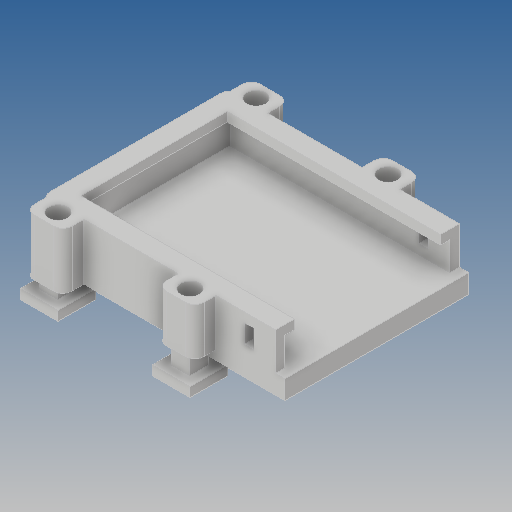
# Autodesk Inventor part: DC-DC корпус
Saved by Autodesk Inventor 2020 (Build 240168000, 168)
## iProperties
Created: 2020-03-21
Part Number: DC-DC корпус
Material: Типовые
Document SubType Name: Modeling
Designer: Iliga
Density: 1 g/cm^3
Appearance: По умолчанию
Author: Iliga
Autodesk Inventor part; units mm, degrees
ref_plane "YZ Plane" through (0, 0, 0) normal (1, 0, 0) x (0, 1, 0)
ref_plane "XZ Plane" through (0, 0, 0) normal (0, 1, 0) x (-1, 0, 0)
ref_plane "XY Plane" through (0, 0, 0) normal (0, 0, 1) x (1, 0, 0)
sketch "Эскиз1" plane through (0, 0, 0) normal (0, 1, 0) x (-1, 0, 0)
  line L0 (-11.5, 8.75) -> (11.5, 8.75)
  line L1 (11.5, 8.75) -> (11.5, -8.75)
  line L2 (11.5, -8.75) -> (-11.5, -8.75)
  line L3 (-11.5, -8.75) -> (-11.5, 8.75)
  line L4 (-11.5, 8.75) -> (11.5, -8.75) construction
  line L5 (11.5, 8.75) -> (-11.5, -8.75) construction
  line L6 (-12.8143, 9.75) -> (12.8143, 9.75)
  line L7 (12.8143, 9.75) -> (12.8143, -9.75)
  line L8 (12.8143, -9.75) -> (-12.8143, -9.75)
  line L9 (-12.8143, -9.75) -> (-12.8143, 9.75)
  line L10 (-12.8143, 9.75) -> (12.8143, -9.75) construction
  line L11 (12.8143, 9.75) -> (-12.8143, -9.75) construction
  point P0 (0, 0)
  dimension "d0" = 23
  dimension "d1" = 17.5
  dimension "d2" = 1
  constraints: 24 end point, 4 midpoint, 4 parallel, 2 horizontal, 2 perpendicular, 1 point on line
  measures "d0" distance of L1.end L2.end
  measures "d1" distance of L0.end L1.end
  measures "d2" distance between parallel lines of L8 L2
extrude "Выдавливание1" add sketch "Эскиз1" against normal blind 1 contours L0 L1 L2 L3 | L6 L7 L8 L9
extrude "Выдавливание2" add sketch "Эскиз1" along normal blind 3
sketch "Эскиз2" plane through (0, 3, 0) normal (0, 1, 0) x (1, 0, 0)
  line L0 (-12.8143, 9.75) -> (-12.8143, -9.75) projected
  line L1 (12.8143, 9.75) -> (-12.8143, 9.75) projected
  line L2 (12.8143, -9.75) -> (12.8143, 9.75) projected
  line L3 (-12.8143, -9.75) -> (12.8143, -9.75) projected
  line L4 (10.8143, -7.75) -> (-10.8143, -7.75)
  line L5 (-10.8143, -7.75) -> (-10.8143, 7.75)
  line L6 (-10.8143, 7.75) -> (10.8143, 7.75)
  line L7 (10.8143, 7.75) -> (10.8143, -7.75)
  line L8 (10.8143, -7.75) -> (-10.8143, 7.75) construction
  line L9 (-10.8143, -7.75) -> (10.8143, 7.75) construction
  point P0 (0, 0)
  dimension "d7" = 2
  dimension "d8" = 2
  constraints: 12 end point, 2 midpoint, 2 parallel, 1 horizontal, 1 perpendicular
  measures "d7" distance between parallel lines of L1 L6
  measures "d8" distance between parallel lines of L0 L5
extrude "Выдавливание3" add sketch "Эскиз2" along normal blind 1
sketch "Эскиз3" plane through (0, 4, 0) normal (0, 1, 0) x (1, 0, 0)
  line L0 (12.8143, -9.75) -> (12.8143, 9.75) projected
  line L1 (11.5, -8.75) -> (11.5, 8.75) projected
  line L2 (10.8143, 7.75) -> (10.8143, -7.75) projected
  line L3 (10.8143, -7.75) -> (11.5, -7.75)
  line L4 (10.8143, 7.75) -> (11.5, 7.75)
  line L5 (11.5, 7.75) -> (11.8143, 7.75)
  line L6 (11.8143, 7.75) -> (11.8143, 9.75)
  line L7 (12.8143, -9.75) -> (11.8143, -9.75)
  line L8 (11.8143, -9.75) -> (11.8143, -7.75)
  line L9 (11.8143, -7.75) -> (11.5, -7.75)
  line L10 (11.8143, 9.75) -> (12.8143, 9.75)
  point P0 (0, 0)
  dimension "d19" = 1
  constraints: 16 end point, 4 horizontal, 3 perpendicular, 2 point on line, 1 vertical alignment
  measures "d19" distance between parallel lines of L0 L6
extrude "Выдавливание4" cut sketch "Эскиз3" against normal up to surface (4 mm away)
sketch "Эскиз5" plane through (-12.8143, -1, 9.75) normal (0, 0, 1) x (1, 0, 0)
  line L0 (24.3143, 1) -> (24.3143, 5) projected
  line L1 (21.3143, 2) -> (22.3143, 2)
  line L2 (22.3143, 2) -> (22.3143, 4)
  line L3 (22.3143, 4) -> (21.3143, 4)
  line L4 (21.3143, 4) -> (21.3143, 2)
  line L5 (21.3143, 2) -> (22.3143, 4) construction
  line L6 (22.3143, 2) -> (21.3143, 4) construction
  point P0 (12.8143, 1)
  point P1 (21.8143, 3)
  point P2 (21.8143, 3)
  point P3 (24.3143, 3)
  dimension "d14" = 2
  dimension "d15" = 2
  dimension "d16" = 1
  constraints: 12 end point, 4 midpoint, 2 parallel, 1 horizontal, 1 horizontal alignment, 1 perpendicular
  measures "d14" distance between parallel lines of L3 L1
  measures "d15" distance between parallel lines of L0 L2
  measures "d16" distance between parallel lines of L4 L2
extrude "Выдавливание5" cut sketch "Эскиз5" against normal up to surface (19.5 mm away)
sketch "Эскиз6" plane through (11.8143, 4, 9.75) normal (1, 0, 0) x (0, 0, -1)
  line L0 (1, -4) -> (1, -1) projected
  line L1 (2, -1) -> (2, -4) projected
  line L2 (1, -4) -> (2, -4) projected
  line L3 (1, -4) -> (1, -1) projected
  line L4 (2, -1) -> (1, -1) projected
  line L5 (17.5, -4) -> (17.5, -1) projected
  line L6 (18.5, -1) -> (17.5, -1) projected
  line L7 (18.5, -4) -> (18.5, -1) projected
  line L8 (17.5, -4) -> (18.5, -4) projected
  point P0 (9.75, -4)
extrude "Выдавливание6" cut sketch "Эскиз6" against normal up to surface (0.3143 mm away)
sketch "Эскиз7" plane through (0, 4, 0) normal (0, 1, 0) x (1, 0, 0)
  line L0 (11.8143, -7.75) -> (-10.8143, -7.75) projected
  line L1 (-10.8143, -7.75) -> (-10.8143, 7.75) projected
  line L2 (-10.8143, 7.75) -> (11.8143, 7.75) projected
  line L3 (11.8143, 7.75) -> (11.8143, 9.75) projected
  line L4 (11.8143, 9.75) -> (-12.8143, 9.75) projected
  line L5 (-12.8143, 9.75) -> (-12.8143, -9.75) projected
  line L6 (-12.8143, -9.75) -> (11.8143, -9.75) projected
  line L7 (11.8143, -9.75) -> (11.8143, -7.75) projected
  line L8 (-12.8143, 9.75) -> (-8.4993, 9.75)
  circle A0 centre (-10.4993, 10.5) radius 1
  line L9 (-12.4993, 12) -> (-12.4993, 9.75)
  line L10 (-8.4993, 9.75) -> (-8.4993, 12)
  line L11 (-8.4993, 12) -> (-12.4993, 12)
  point P0 (0, 0)
  point P1 (-10.4993, 12)
  dimension "d25" = 2
  dimension "d32" = 0.315
  dimension "d52" = 0.75
  dimension "d53" = 1.5
  dimension "d54" = 4
  constraints: 8 end point, 2 perpendicular, 1 centre point, 1 horizontal, 1 midpoint, 1 point on line, 1 vertical, 1 vertical alignment
  measures "d25" diameter of A0
  measures "d32" distance from line of L4.end L9
  measures "d52" distance from line of L4 A0.centre
  measures "d53" distance from line of L11 A0.centre
  measures "d54" distance between parallel lines of L10 L9
extrude "Выдавливание7" add sketch "Эскиз7" against normal up to surface (5 mm away) contours L9 L11 L10 L4 A0
fillet "Сопряжение1" radius 1 2 edges at (-12.4993, 1.5, -12) (-8.4993, 1.5, -12)
sketch "Эскиз8" plane through (0, -1, 0) normal (0, -1, 0) x (1, 0, 0)
  circle A0 centre (-10.4993, -10.5) radius 1 construction
  line L0 (-12.4993, -11) -> (-12.4993, -9.75) projected
  arc A1 (-12.4993, -11) -> (-11.4993, -12) centre (-11.4993, -11) ccw projected
  line L1 (-8.4993, -9.75) -> (12.8143, -9.75) projected
  line L2 (12.8143, -9.75) -> (12.8143, 9.75) projected
  line L3 (12.8143, 9.75) -> (-12.8143, 9.75) projected
  line L4 (-12.8143, 9.75) -> (-12.8143, -9.75) projected
  arc A2 (-11.1607, -9.75) -> (-9.8378, -9.75) centre (-10.4993, -10.5) ccw projected
  line L5 (-8.4993, -9.75) -> (-12.4993, -9.75)
  line L6 (-9.4993, -9.5) -> (-11.4993, -9.5)
  line L7 (-11.4993, -9.5) -> (-11.4993, -11.5)
  line L8 (-11.4993, -11.5) -> (-9.4993, -11.5)
  line L9 (-9.4993, -11.5) -> (-9.4993, -9.5)
  line L10 (-9.4993, -9.5) -> (-11.4993, -11.5) construction
  line L11 (-11.4993, -9.5) -> (-9.4993, -11.5) construction
  line L12 (-12.8143, -9.75) -> (-12.4993, -9.75) projected
  line L13 (-9.4993, -12) -> (-11.4993, -12) projected
  line L14 (-8.4993, -9.75) -> (-8.4993, -11) projected
  line L15 (-11.1607, -9.75) -> (-9.8378, -9.75) projected
  arc A3 (-9.4993, -12) -> (-8.4993, -11) centre (-9.4993, -11) ccw projected
  point P0 (0, 0)
  dimension "d40" = 2
  dimension "d41" = 2
  constraints: 14 end point, 2 horizontal, 2 midpoint, 2 parallel, 1 perpendicular
  measures "d40" distance of L8.end L7.end
  measures "d41" distance of L7.end L6.end
extrude "Выдавливание8" add sketch "Эскиз8" along normal blind 1
extrude "Выдавливание9" add sketch "Эскиз8" along normal blind 2 contours L7 L6 L9 L5 | L5 A2 L7 | L5 A2 | A2 L8 L7 | L5 L9 A2 | A2 L9 L8
sketch "Эскиз9" plane through (0, -3, 0) normal (0, -1, 0) x (1, 0, 0)
  line L0 (-9.4993, -9.5) -> (-11.4993, -9.5) projected
  line L1 (-11.4993, -9.5) -> (-11.4993, -11.5) projected
  line L2 (-11.4993, -11.5) -> (-9.4993, -11.5) projected
  line L3 (-9.4993, -11.5) -> (-9.4993, -9.5) projected
  line L4 (-9.4993, -10.5) -> (-11.4993, -10.5) construction
  line L5 (-8.4993, -8.5) -> (-12.4993, -8.5)
  line L6 (-12.4993, -8.5) -> (-12.4993, -12.5)
  line L7 (-12.4993, -12.5) -> (-8.4993, -12.5)
  line L8 (-8.4993, -12.5) -> (-8.4993, -8.5)
  line L9 (-8.4993, -8.5) -> (-12.4993, -12.5) construction
  line L10 (-12.4993, -8.5) -> (-8.4993, -12.5) construction
  point P0 (0, 0)
  point P1 (-10.4993, -10.5)
  dimension "d44" = 4
  dimension "d45" = 4
  constraints: 14 end point, 5 midpoint, 2 parallel, 1 horizontal, 1 perpendicular
  measures "d44" distance of L7.end L6.end
  measures "d45" distance of L6.end L5.end
extrude "Выдавливание10" add sketch "Эскиз9" along normal blind 1 contours L3 L2 L1 L0 | L8 L7 L6 L5
pattern_linear "Прямоуг.массив2" count 2 spacing 14 along (1, 0, 0) of "Выдавливание7", "Сопряжение1", "Выдавливание9", "Выдавливание10"
mirror "Зеркальное отражение2" about plane through (0, 0, 0) normal (0, 0, 1) of "Выдавливание7", "Сопряжение1", "Выдавливание8", "Выдавливание9", "Выдавливание10", "Прямоуг.массив2"
fillet "Сопряжение3" radius 1 2 edges at (-12.8143, 1, -9.75) (-12.8143, 1, 9.75)
sketch "Эскиз10" plane through (0, 4, 0) normal (0, 1, 0) x (1, 0, 0)
  arc A0 (-9.8378, 9.75) -> (-11.1607, 9.75) centre (-10.4993, 10.5) ccw projected
  circle A1 centre (-10.4993, 10.5) radius 1
  arc A2 (2.8393, -9.75) -> (4.1622, -9.75) centre (3.5007, -10.5) ccw projected
  arc A3 (-11.1607, -9.75) -> (-9.8378, -9.75) centre (-10.4993, -10.5) ccw projected
  arc A4 (4.1622, 9.75) -> (2.8393, 9.75) centre (3.5007, 10.5) ccw projected
  circle A5 centre (3.5007, 10.5) radius 1
  circle A6 centre (3.5007, -10.5) radius 1
  circle A7 centre (-10.4993, -10.5) radius 1
  point P0 (0, 0)
  constraints: 4 coincident, 12 other
extrude "Выдавливание11" cut sketch "Эскиз10" against normal up to surface (5 mm away)
